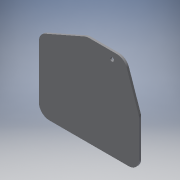
# Autodesk Inventor part: Bucket - door 2
Saved by Autodesk Inventor 2016 (Build 200138000, 138)
## iProperties
Created: 2016-01-14
Part Number: Bucket - door 2
Material: Generic
Document SubType Name: Modeling
Designer: TimB
Density: 1 g/cm^3
Appearance: Default
Author: TimB
Autodesk Inventor part; units mm, degrees
ref_plane "YZ Plane" through (0, 0, 0) normal (1, 0, 0) x (0, 1, 0)
ref_plane "XZ Plane" through (0, 0, 0) normal (0, 1, 0) x (-1, 0, 0)
ref_plane "XY Plane" through (0, 0, 0) normal (0, 0, 1) x (1, 0, 0)
sketch "Sketch1" plane through (0, 0, 0) normal (0, 0, 1) x (1, 0, 0)
  line L0 (72.4944, 63.4773) -> (-72.5056, 63.4773)
  line L1 (72.4944, 63.4773) -> (-72.5232, -63.5025) construction
  line L2 (-72.5056, 63.4773) -> (72.5218, -63.4915) construction
  circle A0 centre (33.08, -58.41) radius 2.85 projected
  line L3 (-72.5056, -38.1227) -> (-3.32, -68.51)
  line L4 (-72.5056, 63.4773) -> (-72.5056, -38.1227)
  line L5 (72.4944, 63.4773) -> (72.4944, -6.5227)
  line L6 (51.23, -68.51) -> (72.4944, -6.5227)
  line L7 (-3.32, -68.51) -> (51.23, -68.51)
  point P0 (0, 0)
  dimension "d6" = 145
  dimension "d9" = 70
  constraints: 16 end point, 2 horizontal, 2 point on line, 1 vertical, 1 other
  measures "d6" distance of L0.start L0.end
  measures "d9" distance of L0.start L5.end
extrude "Extrusion2" add sketch "Sketch1" along normal blind 3
fillet "Fillet1" radius 15 6 edges at (51.23, -68.51, 1.5) (-3.32, -68.51, 1.5) (-72.5056, -38.1227, 1.5) (-72.5056, 63.4773, 1.5) (72.4944, 63.4773, 1.5) (72.4944, -6.5227, 1.5)
body "Solid2"
